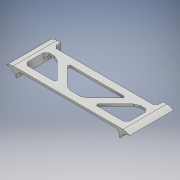
# Autodesk Inventor part: zenter
Saved by Autodesk Inventor 2018 (Build 220112000, 112)
## iProperties
Created: 2019-10-10
Part Number: zenter
Material: Типовые
Document SubType Name: Modeling
Designer: Professional
Density: 1 g/cm^3
Appearance: По умолчанию
Author: Professional
Autodesk Inventor part; units mm, degrees
ref_plane "YZ Plane" through (0, 0, 0) normal (1, 0, 0) x (0, 1, 0)
ref_plane "XZ Plane" through (0, 0, 0) normal (0, 1, 0) x (-1, 0, 0)
ref_plane "XY Plane" through (0, 0, 0) normal (0, 0, 1) x (1, 0, 0)
sketch "Эскиз1" plane through (0, 0, 0) normal (0, 0, 1) x (1, 0, 0)
  line L0 (-70, 0) -> (70, 0)
  line L1 (70, 0) -> (70, 10)
  line L2 (70, 10) -> (-70, 10)
  line L3 (-70, 10) -> (-70, 0)
  line L4 (-70, 0) -> (-84, 0)
  line L5 (-84, 0) -> (-84, 60)
  line L6 (-84, 60) -> (-70, 60)
  line L7 (-70, 60) -> (-70, 0)
  line L8 (-70, 50) -> (-70, 60)
  line L9 (-70, 40) -> (70, 40)
  line L10 (70, 40) -> (70, 50)
  line L11 (70, 50) -> (-70, 50)
  line L12 (-70, 50) -> (-70, 40)
  line L13 (70, 0) -> (84, 0)
  line L14 (84, 0) -> (84, 60)
  line L15 (84, 60) -> (70, 60)
  line L16 (70, 60) -> (70, 0)
  line L17 (-55, 40) -> (-25, 10)
  line L18 (-40.8579, 40) -> (-10.8579, 10)
  line L19 (55, 40) -> (25, 10)
  line L20 (10.8579, 10) -> (40.8579, 40)
  point P0 (0, 0)
  dimension "d0" = 140
  dimension "d1" = 10
  dimension "d2" = 60
  dimension "d4" = 10
  dimension "d5" = 10
  dimension "d6" = 60
  dimension "d7" = 14
  dimension "d8" = 14
  dimension "d9" = 0
  dimension "d24" = 45
  dimension "d25" = 45
  dimension "d26" = 10
  dimension "d27" = 0
  dimension "d28" = 15
  dimension "d29" = 70
  dimension "d30" = 45
  dimension "d31" = 45
  dimension "d32" = 15
  dimension "d33" = 10
  constraints: 42 end point, 9 point on line, 8 parallel, 4 horizontal, 4 perpendicular
  measures "d0" distance of L0.start L0.end
  measures "d1" distance between parallel lines of L0 L2
  measures "d2" distance between parallel lines of L4 L6
  measures "d4" distance between parallel lines of L6 L11
  measures "d5" distance between parallel lines of L9 L11
  measures "d6" distance between parallel lines of L13 L15
  measures "d7" distance between parallel lines of L16 L14
  measures "d8" distance of L0.start L4.end
  measures "d9" distance between parallel lines of L16 L10
  measures "d24" angle of L9 L17
  measures "d25" angle of L9 L18
  measures "d26" distance from line of L18 L17.start
  measures "d27" distance from line of point (0, 0) L0
  measures "d28" distance of L9.start L17.start
  measures "d29" distance from line of point (0, 0) L1
  measures "d30" angle of L9 L19
  measures "d31" angle of L9 L20
  measures "d32" distance from line of L16 L19.start
  measures "d33" distance from line of L19 L20.end
extrude "Выдавливание1" add sketch "Эскиз1" against normal blind 3 contours L3 L2 L1 L0 | L4 L5 L6 L7 L3 | L1 L16 L10 L15 L14 L13 | L17 L9 L18 L2 | L7 L11 L10 L9 | L2 L20 L9 L19
sketch "Эскиз2" plane through (0, 0, -3) normal (0, 0, -1) x (-1, 0, 0)
  line L0 (-70, 60) -> (-84, 60) projected
  line L1 (-70, 60) -> (-71, 60)
  line L2 (-71, 60) -> (-71, 0)
  line L3 (-71, 0) -> (-70, 0)
  line L4 (-70, 0) -> (-70, 60)
  line L5 (70, 60) -> (71, 60)
  line L6 (71, 60) -> (71, 0)
  line L7 (71, 0) -> (70, 0)
  line L8 (70, 0) -> (70, 60)
  line L9 (-84, 0) -> (84, 0) projected
  point P0 (0, 0)
  dimension "d12" = 1
  dimension "d13" = 1
  dimension "d34" = 0
  constraints: 16 end point, 4 parallel, 2 horizontal, 2 perpendicular, 1 point on line
  measures "d12" distance between parallel lines of L4 L2
  measures "d13" distance between parallel lines of L8 L6
  measures "d34" distance between parallel lines of L9 L3
extrude "Выдавливание2" add sketch "Эскиз2" along normal blind 9
fillet "Сопряжение1" radius 13 2 edges at (71, 30, -3) (-71, 30, -3)
chamfer "Фаска2" distance 4 angle 45 14 edges at (-70, 50, -1.5) (-70, 10, -1.5) (-70, 40, -1.5) (70, 10, -1.5) (70, 40, -1.5) (70, 50, -1.5) (25, 10, -1.5) (-10.8579, 10, -1.5) (40.8579, 40, -1.5) (-25, 10, -1.5) (10.8579, 10, -1.5) (-40.8579, 40, -1.5) (-55, 40, -1.5) (55, 40, -1.5)
chamfer "Фаска3" distance 4 angle 45 8 edges at (-70, 52, -3) (-70, 38, -3) (-70, 5, -3) (-70, 12, -3) (70, 52, -3) (70, 38, -3) (70, 5, -3) (70, 12, -3)
fillet "Сопряжение2" radius 15 2 edges at (-84, 30, 0) (84, 30, 0)
